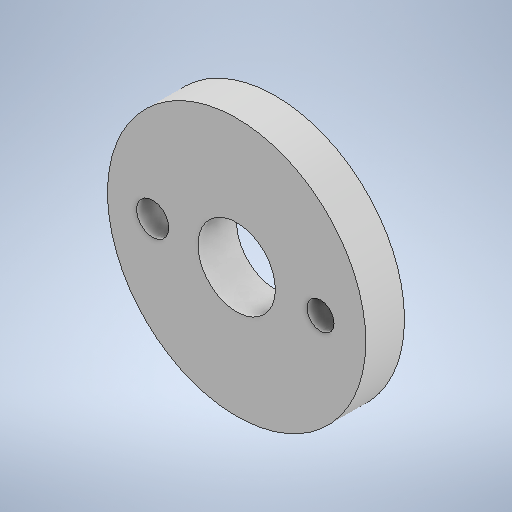
# Autodesk Inventor part: set_6_20
Saved by Autodesk Inventor 2025.1 (Build 291241000, 241)
## iProperties
Created: 2025-05-06
Part Number: set_6_20
Material: 一般
Document SubType Name: Modeling
Designer: yuki0520
Density: 1 g/cm^3
Appearance: 既定
Author: yuki0520
Autodesk Inventor part; units mm, degrees
ref_plane "YZ Plane" through (0, 0, 0) normal (1, 0, 0) x (0, 1, 0)
ref_plane "XZ Plane" through (0, 0, 0) normal (0, 1, 0) x (-1, 0, 0)
ref_plane "XY Plane" through (0, 0, 0) normal (0, 0, 1) x (1, 0, 0)
sketch "スケッチ1" plane through (0, 0, 0) normal (0, 0, 1) x (1, 0, 0)
  circle A0 centre (0, 0) radius 3
  circle A1 centre (0, 0) radius 10
  circle A2 centre (0, 0) radius 6.5
  circle A3 centre (6.5, 0) radius 1.05
  circle A4 centre (-6.5, 0) radius 1.25
  line L0 (-3, 0) -> (3, 0)
  dimension "d0" = 6
  dimension "d1" = 20
  dimension "d2" = 13
  dimension "d3" = 2.1
  dimension "d4" = 2.5
  constraints: 5 centre point, 4 point on circle, 3 coincident, 2 end point, 2 point on line, 1 horizontal, 1 midpoint
  measures "d0" diameter of A0
  measures "d1" diameter of A1
  measures "d2" diameter of A2
  measures "d3" diameter of A3
  measures "d4" diameter of A4
extrude "押し出し1" add sketch "スケッチ1" along normal blind 3 contours A1 | A3 A2 A4
